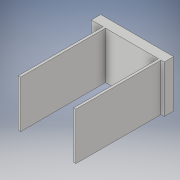
# Autodesk Inventor part: ChainWheelSubAssemblyMainConnector
Saved by Autodesk Inventor 2017 (Build 210142000, 142)
## iProperties
Created: 2017-11-22
Part Number: ChainWheelSubAssemblyMainConnector
Material: Generic
Document SubType Name: Modeling
Designer: User
Density: 1 g/cm^3
Appearance: Default
Author: User
Autodesk Inventor part; units mm, degrees
ref_plane "YZ Plane" through (0, 0, 0) normal (1, 0, 0) x (0, 1, 0)
ref_plane "XZ Plane" through (0, 0, 0) normal (0, 1, 0) x (-1, 0, 0)
ref_plane "XY Plane" through (0, 0, 0) normal (0, 0, 1) x (1, 0, 0)
sketch "Sketch1" plane through (0, 0, 0) normal (0, 0, 1) x (1, 0, 0)
  line L0 (0, 0) -> (98.171, 0)
  line L1 (98.171, 0) -> (98.171, -63.5)
  line L2 (98.171, -63.5) -> (0, -63.5)
  line L3 (0, -63.5) -> (0, 0)
  dimension "d0" = 98.171
  dimension "d1" = 63.5
  constraints: 8 end point, 2 parallel, 1 horizontal, 1 perpendicular
  measures "d0" distance of L1.end L2.end
  measures "d1" distance of L0.end L1.end
extrude "Extrusion1" add sketch "Sketch1" along normal blind 12.7
sketch "Sketch2" plane through (0, 0, 12.7) normal (0, 0, 1) x (1, 0, 0)
  line L0 (0, -63.5) -> (98.171, -63.5) projected
  line L1 (98.171, -63.5) -> (90.551, -63.5)
  line L2 (90.551, -63.5) -> (93.726, -63.5)
  line L3 (93.726, -63.5) -> (93.726, 0)
  line L4 (93.726, 0) -> (90.551, 0)
  line L5 (90.551, 0) -> (90.551, -63.5)
  point P0 (0, 0)
  dimension "d4" = 7.62
  dimension "d5" = 3.175
  constraints: 10 end point, 2 parallel, 1 horizontal, 1 perpendicular, 1 point on line
  measures "d4" distance of L0.end L1.end
  measures "d5" distance of L4.end L3.end
extrude "Extrusion2" add sketch "Sketch2" along normal blind 114.3
sketch "Sketch3" plane through (0, 0, 12.7) normal (0, 0, 1) x (1, 0, 0)
  line L0 (0, 0) -> (15.875, 0)
  line L1 (90.551, 0) -> (0, 0) projected
  line L2 (0, -63.5) -> (90.551, -63.5) projected
  line L3 (15.875, 0) -> (19.05, 0)
  line L4 (19.05, 0) -> (19.05, -63.5)
  line L5 (19.05, -63.5) -> (15.875, -63.5)
  line L6 (15.875, -63.5) -> (15.875, 0)
  dimension "d8" = 15.875
  dimension "d9" = 3.175
  constraints: 10 end point, 2 parallel, 2 point on line, 1 horizontal, 1 perpendicular
  measures "d8" distance of L0.start L0.end
  measures "d9" distance of L4.end L5.end
extrude "Extrusion3" add sketch "Sketch3" along normal blind 114.3
body "Solid1"
